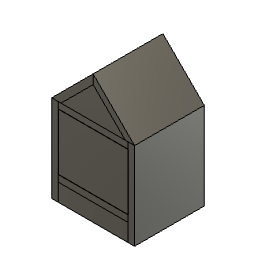
Garduino Housing v2 (Autodesk Fusion 360 design; units mm, degrees)
Autodesk Fusion 360 part; units mm, degrees
sketch "Sketch1" plane through (0, 0, 0) normal (0, 0, 1) x (1, 0, 0)
  line L0 (0, 0) -> (203.2, 0)
  line L1 (203.2, 0) -> (203.2, 19.05)
  line L2 (203.2, 19.05) -> (0, 19.05)
  line L3 (0, 19.05) -> (0, 0)
  line L4 (0, 19.05) -> (203.2, 19.05)
  line L5 (203.2, 19.05) -> (203.2, 184.15)
  line L6 (203.2, 184.15) -> (0, 184.15)
  line L7 (0, 184.15) -> (0, 19.05)
  line L8 (0, 184.15) -> (203.2, 184.15)
  line L9 (203.2, 184.15) -> (203.2, 203.2)
  line L10 (203.2, 203.2) -> (0, 203.2)
  line L11 (0, 203.2) -> (0, 184.15)
  line L12 (0, 203.2) -> (-19.05, 203.2)
  line L13 (-19.05, 203.2) -> (-19.05, 0)
  line L14 (-19.05, 0) -> (0, 0)
  line L15 (0, 0) -> (0, 203.2)
  line L16 (203.2, 203.2) -> (222.25, 203.2)
  line L17 (222.25, 203.2) -> (222.25, 0)
  line L18 (222.25, 0) -> (203.2, 0)
  line L19 (203.2, 0) -> (203.2, 203.2)
  line L20 (101.6, 0) -> (101.6, 450) construction
  line L21 (-19.05, 203.2) -> (101.6, 323.85)
  line L22 (-19.05, 203.2) -> (151.5749, 203.2) construction
  line L23 (222.25, 203.2) -> (101.6, 323.85)
  line L24 (-5.5796, 189.7296) -> (101.6, 296.9092)
  line L25 (208.7796, 189.7296) -> (101.6, 296.9092)
  line L26 (101.6, 323.85) -> (101.6, 295)
  dimension "d1" = 203.2
  dimension "d2" = 19.05
  dimension "d3" = 203.2
  dimension "d4" = 165.1
  dimension "d5" = 203.2
  dimension "d6" = 19.05
  dimension "d7" = 19.05
  dimension "d8" = 19.05
  dimension "d9" = 203.2
  dimension "d23" = 45
  dimension "d24" = 19.05
  constraint horizontal L0
  constraint vertical L1
  constraint horizontal L2
  constraint vertical L3
  constraint coincident L0.start L3.end
  constraint horizontal L4
  constraint vertical L5
  constraint horizontal L6
  constraint vertical L7
  constraint horizontal L8
  constraint vertical L9
  constraint horizontal L10
  constraint vertical L11
  constraint horizontal L12
  constraint vertical L13
  constraint horizontal L14
  constraint vertical L15
  constraint horizontal L16
  constraint vertical L17
  constraint horizontal L18
  constraint vertical L19
  constraint midpoint L0 L20.start
  constraint perpendicular L2 L20
  constraint horizontal L22
  constraint coincident L20 L21.end
  constraint coincident L20 L26.end
  measures "d1" distance of L0.start L0.end
  measures "d2" distance of L0.start L2.end
  measures "d3" distance of L2.end L1.end
  measures "d4" distance of L2.end L6.end
  measures "d5" distance of L6.end L5.end
  measures "d6" distance of L6.end L10.end
  measures "d7" distance of L10.end L12.end
  measures "d8" distance of L9.end L16.end
  measures "d9" distance of L9.end L0.end
  measures "d23" angle of L21 L22
extrude "Extrude1" add sketch "Sketch1" along normal blind 203.2 contours L3 L7 L11 L12 L13 L14 L15 makes body 1
extrude "Extrude2" add sketch "Sketch1" along normal blind 203.2 separate body contours L1 L5 L9 L16 L17 L18 L19 makes body 2
extrude "Extrude3" add sketch "Sketch1" along normal blind 203.2 separate body contours L6 L8 L9 L10 L11 L15 L19 L24 L25 | L10 L11 L15 L24 | L9 L10 L19 L25 makes body 3
extrude "Extrude4" add sketch "Sketch1" along normal blind 203.2 separate body contours L0 L1 L2 L3 L4 L15 L19 makes body 4
extrude "Extrude5" add sketch "Sketch1" along normal blind 19.05 separate body contours L2 L4 L5 L6 L7 L8 L15 L19 makes body 5
extrude "Extrude6" add sketch "Sketch1" against normal blind 0.75 from surface at 203.2 separate body contours L2 L4 L5 L6 L7 L8 L15 L19 makes body 6
extrude "Extrude7" add sketch "Sketch1" along normal blind 203.2 separate body contours L10 L12 L21 L24 L26 makes body 7
extrude "Extrude8" add sketch "Sketch1" along normal blind 203.2 separate body contours L10 L16 L23 L25 L26 makes body 8
ref_plane "WorkPlane1" through (101.6, 0, 101.6) normal (0, -1, 0) x (1, 0, 0)
sketch "Sketch2" plane through (101.6, 0, 101.6) normal (0, -1, 0) x (1, 0, 0)
  line L0 (-101.6, -101.6) -> (101.6, -101.6)
  line L1 (101.6, -101.6) -> (101.6, 101.6)
  line L2 (101.6, 101.6) -> (-101.6, 101.6)
  line L3 (-101.6, 101.6) -> (-101.6, -101.6)
  line L4 (-120.65, -101.6) -> (-101.6, -101.6)
  line L5 (-101.6, -101.6) -> (-101.6, 101.6)
  line L6 (-101.6, 101.6) -> (-120.65, 101.6)
  line L7 (-120.65, 101.6) -> (-120.65, -101.6)
  line L8 (101.6, -101.6) -> (120.65, -101.6)
  line L9 (120.65, -101.6) -> (120.65, 101.6)
  line L10 (120.65, 101.6) -> (101.6, 101.6)
  line L11 (101.6, 101.6) -> (101.6, -101.6)
  line L12 (-101.6, 101.6) -> (101.6, 101.6)
  line L13 (101.6, 101.6) -> (101.6, 82.55)
  line L14 (101.6, 82.55) -> (-101.6, 82.55)
  line L15 (-101.6, 82.55) -> (-101.6, 101.6)
  line L16 (101.6, -101.6) -> (-101.6, -101.6)
  line L17 (-101.6, -101.6) -> (-101.6, -82.55)
  line L18 (-101.6, -82.55) -> (101.6, -82.55)
  line L19 (101.6, -82.55) -> (101.6, -101.6)
  dimension "d30" = 203.2
  dimension "d31" = 19.05
  dimension "d32" = 203.2
  dimension "d33" = 19.05
  constraint horizontal L12
  constraint vertical L13
  constraint horizontal L14
  constraint vertical L15
  constraint coincident L2.end L3.start
  constraint horizontal L16
  constraint vertical L17
  constraint horizontal L18
  constraint vertical L19
  constraint coincident L0.end L1.start
  measures "d30" distance of L2.end L1.end
  measures "d31" distance of L2.end L14.end
  measures "d32" distance of L0.end L0.start
  measures "d33" distance of L0.end L18.end
extrude "Extrude9" add sketch "Sketch2" along normal blind 50.8 separate body contours L1 L2 L3 L5 L11 L12 L13 L14 L15 makes body 9
extrude "Extrude10" add sketch "Sketch2" along normal blind 50.8 separate body contours L1 L8 L9 L10 L11 L13 L19 makes body 10
extrude "Extrude11" add sketch "Sketch2" along normal blind 50.8 separate body contours L3 L4 L5 L6 L7 L15 L17 makes body 11
extrude "Extrude12" add sketch "Sketch2" along normal blind 50.8 separate body contours L0 L1 L3 L5 L11 L16 L17 L18 L19 makes body 12
combine "Combine1" operation add target body 10 tool bodies 2
combine "Combine2" operation add target body 11 tool bodies 1
extrude "Extrude13" add sketch "Sketch1" along normal blind 19.05 separate body contours L10 L24 L25 makes body 13
extrude "Extrude14" add sketch "Sketch1" against normal blind 19.05 from surface at 203.2 separate body contours L10 L24 L25 makes body 14
sketch "Sketch3" plane through (0, 0, 0) normal (0, -1, 0) x (1, 0, 0)
  line L0 (0, 0) -> (203.2, 0)
  line L1 (203.2, 0) -> (203.2, 203.2)
  line L2 (203.2, 203.2) -> (0, 203.2)
  line L3 (0, 203.2) -> (0, 0)
  line L4 (50.8, 158.75) -> (177.8, 158.75)
  line L5 (177.8, 158.75) -> (177.8, 44.45)
  line L6 (177.8, 44.45) -> (50.8, 44.45)
  line L7 (50.8, 44.45) -> (50.8, 158.75)
  line L8 (0, 184.15) -> (203.2, 184.15)
  dimension "d47" = 127
  dimension "d48" = 114.3
  dimension "d49" = 25.4
  dimension "d50" = 25.4
  constraint horizontal L4
  constraint vertical L5
  constraint horizontal L6
  constraint vertical L7
  measures "d47" distance of L4.start L4.end
  measures "d48" distance of L4.start L6.end
  measures "d49" distance of L4 L8
  measures "d50" distance of L1 L5
extrude "Extrude15" cut sketch "Sketch3" against normal up to surface (19.05 mm away) contours L4 L5 L6 L7 bodies 4
ref_plane "WorkPlane2" through (-19.05, 76.2, 101.6) normal (-1, 0, 0) x (0, 0, -1)
sketch "Sketch4" plane through (-19.05, 76.2, 101.6) normal (-1, 0, 0) x (0, 0, -1)
  line L0 (-101.6, 76.2) -> (-82.55, 76.2)
  line L1 (-101.6, 76.2) -> (106.4059, 76.2) construction
  line L2 (101.6, -127) -> (101.6, 127) construction
  line L3 (101.6, 127) -> (-101.6, 127) construction
  line L4 (-101.6, 127) -> (-101.6, -127) construction
  line L5 (-101.6, -127) -> (101.6, -127) construction
  line L6 (101.6, 57.15) -> (-101.6, 57.15) construction
  line L7 (0, -127) -> (0, 57.15)
  line L8 (101.6, -34.925) -> (-101.6, -34.925)
  line L9 (22.225, -54.61) -> (-22.225, -54.61)
  line L10 (-22.225, -54.61) -> (-22.225, -15.24)
  line L11 (-22.225, -15.24) -> (22.225, -15.24)
  line L12 (22.225, -15.24) -> (22.225, -54.61)
  dimension "d54" = 19.05
  dimension "d55" = 92.075
  dimension "d56" = 44.45
  dimension "d57" = 39.37
  dimension "d58" = 19.685
  dimension "d59" = 22.225
  constraint coincident L0.start L1.start
  constraint parallel L0 L1
  constraint coincident L2 L6.start
  constraint coincident L4 L6.end
  constraint perpendicular L4 L6
  constraint midpoint L5 L7.start
  constraint midpoint L6 L7.end
  constraint coincident L2 L8.start
  constraint coincident L4 L8.end
  constraint perpendicular L4 L8
  constraint horizontal L9
  constraint vertical L10
  constraint horizontal L11
  constraint vertical L12
  measures "d54" distance of L1 L6
  measures "d55" distance of L5 L8
  measures "d56" distance of L9.start L9.end
  measures "d57" distance of L9.start L11.end
  measures "d58" distance of L8 L9
  measures "d59" distance of L7 L12
extrude "Extrude16" cut sketch "Sketch4" against normal up to surface (19.05 mm away) bodies 11
